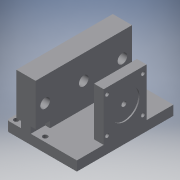
# Autodesk Inventor part: Near Gantry Bracket
Saved by Autodesk Inventor 2016 (Build 200138000, 138)
## iProperties
Created: 2016-04-12
Part Number: Near Gantry Bracket
Material: Generic
Document SubType Name: Modeling
Designer: rubenjm
Density: 1 g/cm^3
Appearance: Default
Author: rubenjm
Autodesk Inventor part; units mm, degrees
ref_plane "YZ Plane" through (0, 0, 0) normal (1, 0, 0) x (0, 1, 0)
ref_plane "XZ Plane" through (0, 0, 0) normal (0, 1, 0) x (-1, 0, 0)
ref_plane "XY Plane" through (0, 0, 0) normal (0, 0, 1) x (1, 0, 0)
sketch "Sketch1" plane through (0, 0, 0) normal (0, 1, 0) x (-1, 0, 0)
  line L0 (3.175, 0) -> (47.625, 0)
  line L1 (50.8, -3.175) -> (50.8, -123.825)
  line L2 (47.625, -127) -> (3.175, -127)
  arc A0 (50.8, -3.175) -> (47.625, 0) centre (47.625, -3.175) ccw
  arc A1 (47.625, -127) -> (50.8, -123.825) centre (47.625, -123.825) ccw
  line L3 (0, 0) -> (-41.656, 0)
  line L4 (-41.656, 0) -> (-41.656, -127)
  line L5 (-41.656, -127) -> (0, -127)
  line L6 (3.175, -127) -> (0, -127)
  line L7 (3.175, 0) -> (0, 0)
  point P0 (50.8, -127)
  point P1 (50.8, 0)
  point P2 (0, -127)
  dimension "d0" = 50.8
  dimension "d1" = 127
  dimension "d4" = 3.175
  dimension "d39" = 41.656
  dimension "d40" = 127
  constraints: 16 end point, 6 point on line, 4 point on circle, 4 tangent, 2 centre point, 2 horizontal, 2 parallel, 2 perpendicular, 1 collinear
  measures "d0" distance of point (50.8, -127) point (0, -127)
  measures "d1" distance of point (50.8, 0) point (50.8, -127)
  measures "d4" radius of A0
  measures "d39" distance of L5.end L4.end
  measures "d40" distance of L4.end L3.end
extrude "Extrusion1" add sketch "Sketch1" along normal blind 12.7
sketch "Sketch2" plane through (0, 12.7, 0) normal (0, 1, 0) x (1, 0, 0)
  line L0 (0, 0) -> (-6.35, 0) construction
  line L1 (-6.35, 0) -> (-6.35, 6.35) construction
  line L2 (-6.35, 6.35) -> (0, 6.35) construction
  line L3 (0, 6.35) -> (0, 0) construction
  circle A0 centre (-6.35, 6.35) radius 3.175
  line L4 (0, 3.175) -> (0, 123.825) construction
  line L5 (0, 63.5) -> (-50.8802, 63.5) construction
  line L6 (-50.8802, 63.5) -> (-25.4, 127) construction
  line L7 (41.656, 127) -> (-47.625, 127) construction
  line L8 (-25.4, 127) -> (-25.4, 0) construction
  line L9 (-47.625, 0) -> (41.656, 0) construction
  circle A1 centre (-6.35, 120.65) radius 3.175
  circle A2 centre (-44.45, 6.35) radius 3.175
  circle A3 centre (-44.45, 120.65) radius 3.175
  point P0 (-3.175, 127)
  point P1 (-3.175, 0)
  dimension "d5" = 6.35
  dimension "d6" = 6.35
  dimension "d7" = 6.35
  constraints: 14 end point, 4 centre point, 3 symmetric about line, 2 horizontal, 2 parallel, 2 point on line, 1 coincident, 1 midpoint, 1 perpendicular, 3 other
  measures "d5" distance of L1.end L2.end
  measures "d6" distance of L0.end L1.end
  measures "d7" diameter of A0
extrude "Extrusion2" cut sketch "Sketch2" against normal through all
sketch "Sketch3" plane through (0, 12.7, 0) normal (0, 1, 0) x (1, 0, 0)
  line L0 (0, 0) -> (-12.7, 0) construction
  line L1 (0, 0) -> (12.7, 0) construction
  line L2 (-47.625, 0) -> (41.656, 0) construction
  line L3 (-25.4, 0) -> (-25.4, 127) construction
  line L4 (41.656, 127) -> (-47.625, 127) construction
  line L5 (-50.8, 0) -> (-38.1, 0) construction
  line L6 (-38.1, 0) -> (-12.7, 0)
  line L7 (-12.7, 0) -> (-12.7, 127)
  line L8 (-12.7, 127) -> (-38.1, 127)
  line L9 (-38.1, 127) -> (-38.1, 0)
  point P0 (-3.175, 0)
  point P1 (-3.175, 127)
  dimension "d14" = 12.7
  dimension "d15" = 180
  dimension "d36" = 25.4
  constraints: 16 end point, 3 horizontal, 3 point on line, 2 parallel, 2 symmetric about line, 1 collinear, 1 perpendicular
  measures "d14" distance of L0.start L0.end
  measures "d15" angle of L0 L1
  measures "d36" distance of L6.end L5.end
extrude "Extrusion3" add sketch "Sketch3" along normal blind 63.5
sketch "Sketch4" plane through (0, 0, 0) normal (0, -1, 0) x (1, 0, 0)
  line L0 (0, 0) -> (-12.7, 0) construction
  line L1 (-12.7, 0) -> (-12.7, -12.7) construction
  line L2 (-12.7, -12.7) -> (0, -12.7) construction
  line L3 (0, -12.7) -> (0, 0) construction
  line L4 (-12.7, -12.7) -> (-38.1, -12.7)
  line L5 (-38.1, -12.7) -> (-38.1, -112.7528)
  line L6 (-38.1, -112.7528) -> (-12.7, -112.7528)
  line L7 (-12.7, -112.7528) -> (-12.7, -12.7)
  dimension "d18" = 12.7
  dimension "d19" = 12.7
  constraints: 16 end point, 4 parallel, 2 horizontal, 2 perpendicular
  measures "d18" distance of L2.end L1.end
  measures "d19" distance of L1.end L0.end
extrude "Extrusion4" cut sketch "Sketch4" against normal blind 6.35
sketch "Sketch5" plane through (-12.7, 12.7, 0) normal (1, 0, 0) x (0, 0, -1)
  line L0 (0, 63.5) -> (127, 63.5) construction
  line L1 (63.5, 63.5) -> (63.5, 0) construction
  line L2 (123.825, 0) -> (3.175, 0) construction
  line L3 (127, 0) -> (127, 63.5) construction
  circle A0 centre (63.4683, 31.7498) radius 6.35
  circle A1 centre (12.6683, 31.7498) radius 6.35
  circle A2 centre (114.2683, 31.7498) radius 6.35
  line L4 (0, 0) -> (0, 63.5) construction
  line L5 (0, 31.75) -> (127, 31.75) construction
  point P0 (0, -12.7)
  dimension "d24" = 12.7
  dimension "d27" = 12.7
  dimension "d37" = 50.8
  dimension "d38" = 50.8
  constraints: 4 end point, 4 midpoint, 3 centre point
  measures "d24" diameter of A0
  measures "d27" diameter of A1
  measures "d37" distance of A1.centre A0.centre
  measures "d38" distance of A2.centre A0.centre
extrude "Extrusion5" cut sketch "Sketch5" against normal through all
sketch "Sketch6" plane through (0, 12.7, 0) normal (0, 1, 0) x (1, 0, 0)
  line L0 (-12.7, 0) -> (-19.05, 0)
  line L1 (-19.05, 0) -> (-19.05, 19.05)
  line L2 (-19.05, 19.05) -> (-12.7, 19.05)
  line L3 (-12.7, 19.05) -> (-12.7, 0)
  line L4 (-38.1, 127) -> (-38.1, 0) construction
  line L5 (-38.4604, 63.7403) -> (-13.0604, 63.7086) construction
  line L6 (-12.7, 69.8183) -> (-12.7, 57.1183) construction
  line L7 (-12.541, 127.416) -> (-18.891, 127.4319)
  line L8 (-18.891, 127.4319) -> (-18.9385, 108.3819)
  line L9 (-18.9385, 108.3819) -> (-12.5885, 108.3661)
  line L10 (-12.5885, 108.3661) -> (-12.541, 127.416)
  line L11 (-47.625, 0) -> (41.656, 0) construction
  line L12 (-25.4, 0) -> (-25.4, 127) construction
  line L13 (41.656, 127) -> (-47.625, 127) construction
  line L14 (-38.1, 0) -> (-31.75, 0)
  line L15 (-31.75, 0) -> (-31.75, 19.05)
  line L16 (-31.75, 19.05) -> (-38.1, 19.05)
  line L17 (-38.1, 19.05) -> (-38.1, 0)
  line L18 (-38.1, 69.8183) -> (-38.1, 57.1183) construction
  line L19 (-38.259, 127.416) -> (-31.909, 127.4319)
  line L20 (-31.909, 127.4319) -> (-31.8615, 108.3819)
  line L21 (-31.8615, 108.3819) -> (-38.2115, 108.3661)
  line L22 (-38.2115, 108.3661) -> (-38.259, 127.416)
  line L23 (-47.625, 0) -> (-2.456, 0) construction
  point P0 (0, 0)
  point P1 (-3.175, 0)
  point P2 (-3.175, 127)
  point P3 (-37.7396, 63.7086)
  point P4 (-38.1, 69.8183)
  point P5 (-38.1, 57.1183)
  dimension "d30" = 6.35
  dimension "d31" = 19.05
  constraints: 38 end point, 15 symmetric about line, 3 point on line, 2 parallel, 1 horizontal, 1 perpendicular, 3 other
  measures "d30" distance of L1.end L2.end
  measures "d31" distance of L0.end L1.end
extrude "Extrusion6" cut sketch "Sketch6" along normal blind 8.382
sketch "Sketch7" plane through (0, 12.7, 0) normal (0, 1, 0) x (1, 0, 0)
  line L0 (41.5616, 127.6536) -> (41.5616, 0) construction
  line L1 (41.656, 0) -> (41.656, 127) projected
  line L2 (41.656, 63.5) -> (28.956, 63.5) construction
  line L3 (28.956, 63.5) -> (28.956, 35.3)
  line L4 (28.956, 35.3) -> (41.656, 35.3)
  line L5 (41.656, 35.3) -> (41.656, 63.5)
  line L6 (28.956, 63.5) -> (28.956, 91.7)
  line L7 (28.956, 91.7) -> (41.656, 91.7)
  line L8 (41.656, 91.7) -> (41.656, 63.5)
  point P0 (0, 0)
  dimension "d41" = 12.7
  dimension "d42" = 28.2
  constraints: 16 end point, 2 parallel, 2 symmetric about line, 1 horizontal, 1 midpoint, 1 perpendicular, 1 vertical
  measures "d41" distance of L4.end L3.end
  measures "d42" distance of L3.end L2.end
extrude "Extrusion7" add sketch "Sketch7" along normal blind 63.5
sketch "Sketch8" plane through (41.656, 0, 0) normal (1, 0, 0) x (0, 0, -1)
  line L0 (127, 0) -> (123.825, 0) construction
  line L1 (0, 0) -> (127, 0) construction
  line L2 (123.825, 0) -> (3.175, 0) construction
  line L3 (63.5, 0) -> (63.5, 13.8176) construction
  circle A0 centre (63.4683, 44.4498) radius 6.35 construction
  line L4 (63.5, 13.8176) -> (63.4683, 44.4498) construction
  circle A1 centre (63.4683, 44.4498) radius 19.05
  dimension "d45" = 13.8176
  dimension "d46" = 38.1
  constraints: 6 end point, 1 centre point, 1 coincident, 1 horizontal, 1 midpoint, 1 vertical
  measures "d45" distance of L3.start L3.end
  measures "d46" diameter of A1
extrude "Extrusion8" cut sketch "Sketch8" against normal blind 1.6
sketch "Sketch9" plane through (41.656, 0, 0) normal (1, 0, 0) x (0, 0, -1)
  line L0 (127, 0) -> (123.825, 0) construction
  line L1 (0, 0) -> (127, 0) construction
  line L2 (123.825, 0) -> (3.175, 0) construction
  line L3 (63.5, 0) -> (63.5, 13.8176) construction
  circle A0 centre (63.4683, 44.4498) radius 3.25
  line L4 (63.5, 13.8176) -> (63.4683, 44.4498) construction
  circle A1 centre (63.4683, 44.4498) radius 19.05 construction
  dimension "d49" = 13.8176
  dimension "d50" = 38.1
  dimension "d51" = 6.5
  constraints: 10 end point, 2 centre point, 1 coincident, 1 horizontal, 1 midpoint, 1 vertical
  measures "d49" distance of L3.start L3.end
  measures "d50" diameter of A1
  measures "d51" diameter of A0
extrude "Extrusion9" cut sketch "Sketch9" against normal through all
sketch "Sketch10" plane through (41.656, 0, 0) normal (1, 0, 0) x (0, 0, -1)
  line L0 (127, 0) -> (123.825, 0) construction
  line L1 (0, 0) -> (127, 0) construction
  line L2 (123.825, 0) -> (3.175, 0) construction
  line L3 (63.5, 0) -> (63.5, 13.8176) construction
  circle A0 centre (63.4683, 44.4498) radius 6.35 construction
  line L4 (63.5, 13.8176) -> (63.4683, 44.4498) construction
  circle A1 centre (63.4683, 44.4498) radius 19.05 construction
  line L5 (87.0383, 68.0198) -> (39.8983, 68.0198) construction
  line L6 (39.8983, 68.0198) -> (39.8983, 20.8798) construction
  line L7 (39.8983, 20.8798) -> (87.0383, 20.8798) construction
  line L8 (87.0383, 20.8798) -> (87.0383, 68.0198) construction
  circle A2 centre (63.4683, 44.4498) radius 3.25 construction
  line L9 (87.0383, 68.0198) -> (39.8983, 20.8798) construction
  line L10 (39.8983, 68.0198) -> (87.0383, 20.8798) construction
  circle A3 centre (87.0383, 20.8798) radius 2.5
  circle A4 centre (39.8984, 20.8798) radius 2.5
  circle A5 centre (39.8983, 68.0198) radius 2.5
  circle A6 centre (87.0383, 68.0198) radius 2.5
  dimension "d54" = 13.8176
  dimension "d55" = 38.1
  dimension "d56" = 47.14
  dimension "d57" = 47.14
  dimension "d58" = 5
  dimension "d59" = 5
  dimension "d60" = 5
  dimension "d61" = 5
  constraints: 22 end point, 6 centre point, 3 midpoint, 2 coincident, 2 horizontal, 2 parallel, 1 perpendicular, 1 vertical
  measures "d54" distance of L3.start L3.end
  measures "d55" diameter of A1
  measures "d56" distance of L7.end L6.end
  measures "d57" distance of L6.end L5.end
  measures "d58" diameter of A3
  measures "d59" diameter of A4
  measures "d60" diameter of A5
  measures "d61" diameter of A6
extrude "Extrusion10" cut sketch "Sketch10" against normal up to surface (12.7 mm away)
body "Solid1"
